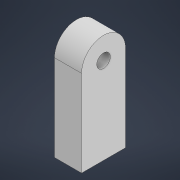
# Autodesk Inventor part: gear support
Saved by Autodesk Inventor 2022 (Build 260153000, 153)
## iProperties
Created: 2022-01-25
Part Number: gear support
Material: Generic
Document SubType Name: Modeling
Designer: gordo
Density: 1 g/cm^3
Appearance: Default
Author: gordo
Autodesk Inventor part; units mm, degrees
ref_plane "YZ Plane" through (0, 0, 0) normal (1, 0, 0) x (0, 1, 0)
ref_plane "XZ Plane" through (0, 0, 0) normal (0, 1, 0) x (-1, 0, 0)
ref_plane "XY Plane" through (0, 0, 0) normal (0, 0, 1) x (1, 0, 0)
sketch "Sketch1" plane through (0, 0, 0) normal (0, 1, 0) x (-1, 0, 0)
  line L0 (0, 0) -> (12.7, 0)
  line L1 (12.7, 0) -> (12.7, -25.4)
  line L2 (12.7, -25.4) -> (0, -25.4)
  line L3 (0, -25.4) -> (0, 0)
  dimension "d1" = 25.4
  dimension "d2" = 12.7
  constraints: 8 end point, 2 parallel, 1 horizontal, 1 perpendicular
  measures "d1" distance between parallel lines of L2 L0
  measures "d2" distance between parallel lines of L3 L1
extrude "Extrusion1" add sketch "Sketch1" along normal blind 45
sketch "Sketch7" plane through (0, 45, 0) normal (0, 1, 0) x (1, 0, 0)
  line L0 (-12.7, 0) -> (0, 0) projected
  line L1 (-12.7, 25.4) -> (-12.7, 0) projected
  line L2 (0, 0) -> (-12.7, 0)
  line L3 (-12.7, 0) -> (-12.7, 25.4)
  line L4 (-12.7, 25.4) -> (0, 25.4)
  line L5 (0, 25.4) -> (0, 0)
  constraints: 8 end point, 2 parallel, 1 horizontal, 1 perpendicular
extrude "Extrusion6" add sketch "Sketch7" along normal blind 15
sketch "Sketch12" plane through (0, 60, 0) normal (0, 1, 0) x (1, 0, 0)
  line L0 (0, 0) -> (0, 25.4) projected
  line L1 (-12.7, 25.4) -> (-12.7, 0) projected
  line L2 (0, 4.8) -> (-12.7, 4.8)
  line L3 (-12.7, 4.8) -> (-12.7, 25.4)
  line L4 (-12.7, 25.4) -> (0, 25.4)
  line L5 (0, 25.4) -> (0, 4.8)
  point P0 (-12.7, 4.8)
  point P1 (-12.7, 4.8)
  constraints: 8 end point, 2 parallel, 1 horizontal, 1 perpendicular
extrude "Extrusion11" cut sketch "Sketch12" against normal blind 9.216
fillet "Fillet5" radius 10.3 1 edges at (-6.35, 50.784, -25.4)
sketch "Sketch14" plane through (-12.7, 0, 0) normal (0, 0, 1) x (1, 0, 0)
  line L0 (0, 60) -> (12.7, 60) projected
  line L1 (12.7, 0) -> (12.7, 40.484) projected
  line L2 (0, 60) -> (12.7, 60)
  line L3 (12.7, 60) -> (12.7, 0)
  line L4 (12.7, 0) -> (0, 0)
  line L5 (0, 0) -> (0, 60)
  constraints: 8 end point, 2 parallel, 1 horizontal, 1 perpendicular
extrude "Extrusion13" cut sketch "Sketch14" against normal blind 4.8
fillet "Fillet6" radius 10.3 1 edges at (-6.35, 50.784, -4.8)
sketch "Sketch18" plane through (0, 0, -25.4) normal (1, 0, 0) x (0, 0, -1)
  arc A0 (0, 40.484) -> (-20.6, 40.484) centre (-10.3, 40.484) ccw projected
  circle A1 centre (-10.3, 40.484) radius 3.175
  point P0 (-25.4, 0)
  dimension "d65" = 6.35
  constraints: 1 centre point, 1 coincident
  measures "d65" diameter of A1
extrude "Extrusion17" cut sketch "Sketch18" against normal through all
body "Solid1"
